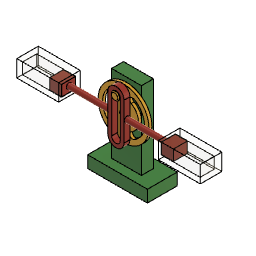
scotch yoke mechanism (piston) (Autodesk Fusion 360 design; units mm, degrees)
Autodesk Fusion 360 part; units mm, degrees
sketch "base" plane through (0, 0, 0) normal (0, 0, 1) x (1, 0, 0)
  line L0 (0, 0) -> (100, 0)
  line L1 (100, 0) -> (100, 50)
  line L2 (100, 50) -> (0, 50)
  line L3 (0, 50) -> (0, 0)
  line L4 (50, 35) -> (75, 35)
  line L5 (75, 35) -> (75, 15)
  line L6 (75, 15) -> (50, 15)
  line L7 (50, 15) -> (50, 35)
  line L8 (50, 35) -> (25, 35)
  line L9 (25, 35) -> (25, 15)
  line L10 (25, 15) -> (50, 15)
  dimension "d1" = 100
  dimension "d2" = 50
  constraint horizontal L0
  constraint vertical L1
  constraint horizontal L2
  constraint vertical L3
  constraint coincident L0.start L3.end
  constraint horizontal L4
  constraint vertical L5
  constraint horizontal L6
  constraint vertical L7
  constraint symmetric L4.start L7 L8.start
  constraint symmetric L4.end L7 L8.end
  constraint symmetric L5.end L7 L9.end
  constraint symmetric L6.end L7 L10.end
  measures "d1" distance of L0.start L0.end
  measures "d2" distance of L0.start L2.end
  measures "d85" distance of L0.start
extrude "Extrude1" add sketch "base" along normal blind 20 makes body 1
extrude "Extrude2" add sketch "base" along normal blind 150 separate body contours L4 L5 L6 L7 | L7 L8 L9 L10 makes body 2
sketch "stand" plane through (0, 15, 0) normal (0, -1, 0) x (1, 0, 0)
  line L0 (25, 0) -> (75, 0)
  line L1 (75, 0) -> (75, 150)
  line L2 (75, 150) -> (25, 150)
  line L3 (25, 150) -> (25, 0)
  circle A0 centre (50, 100) radius 5
  dimension "d7" = 10
  measures "d7" diameter of A0
extrude "Extrude3" add sketch "stand" along normal blind 7 contours A0 bodies 2
sketch "crank" plane through (0, 15, 0) normal (0, -1, 0) x (1, 0, 0)
  circle A0 centre (50, 100) radius 5
  line L0 (25, 0) -> (75, 0)
  line L1 (75, 0) -> (75, 150)
  line L2 (75, 150) -> (25, 150)
  line L3 (25, 150) -> (25, 0)
  circle A1 centre (50, 100) radius 42.5
  dimension "d10" = 85
  constraint concentric A0 A1
  measures "d10" diameter of A1
extrude "Extrude4" add sketch "crank" along normal blind 5 separate body contours L3 A1 | L1 L3 A1 | L1 A1 makes body 3
move_face "OffsetFaces1" offset -0.4 1 faces at (54.9752, 12.6667, 100.4978) on bodies 2
sketch "slots" plane through (0, 10, 0) normal (0, -1, 0) x (1, 0, 0)
  circle A0 centre (50, 100) radius 5
  circle A1 centre (50, 100) radius 42.5
  arc A2 (37.3529, 120.5882) -> (37.3529, 79.4118) centre (48.3333, 100) ccw
  arc A3 (37.3529, 120.5882) -> (32.6471, 129.4118) centre (35, 125) ccw
  arc A4 (32.6471, 129.4118) -> (32.6471, 70.5882) centre (48.3333, 100) ccw
  arc A5 (32.6471, 70.5882) -> (37.3529, 79.4118) centre (35, 75) ccw
  arc A6 (35, 125) -> (35, 75) centre (48.3333, 100) ccw construction
  line L0 (50, 142.5) -> (50, 57.5)
  arc A7 (62.6471, 79.4118) -> (62.6471, 120.5882) centre (51.6667, 100) ccw
  arc A8 (67.3529, 70.5882) -> (67.3529, 129.4118) centre (51.6667, 100) ccw
  arc A9 (67.3529, 129.4118) -> (62.6471, 120.5882) centre (65, 125) ccw
  arc A10 (62.6471, 79.4118) -> (67.3529, 70.5882) centre (65, 75) ccw
  arc A11 (65, 75) -> (65, 125) centre (51.6667, 100) ccw construction
  constraint tangent A2 A3
  constraint tangent A3 A4
  constraint tangent A4 A5
  constraint tangent A2 A5
  constraint coincident A1 L0.start
  constraint coincident A1 L0.end
  constraint vertical L0
  constraint symmetric A2.end L0 A7.start
  constraint symmetric A2.start L0 A7.end
  constraint symmetric A3.end L0 A8.end
  constraint symmetric A4.end L0 A8.start
  constraint symmetric A2 L0 A7
  constraint symmetric A3 L0 A9
  constraint symmetric A4 L0 A8
  constraint symmetric A5 L0 A10
  constraint symmetric A6 L0 A11
extrude "Extrude5" cut sketch "slots" against normal blind 5 contours A2 A3 A4 A5 | A7 A8 A9 A10 bodies 3
sketch "pin" plane through (0, 10, 0) normal (0, -1, 0) x (1, 0, 0)
  arc A0 (32.6471, 129.4118) -> (32.6471, 70.5882) centre (48.3333, 100) ccw
  arc A1 (37.3529, 120.5882) -> (32.6471, 129.4118) centre (35, 125) ccw
  arc A2 (37.3529, 120.5882) -> (37.3529, 79.4118) centre (48.3333, 100) ccw
  arc A3 (32.6471, 70.5882) -> (37.3529, 79.4118) centre (35, 75) ccw
  arc A4 (67.3529, 70.5882) -> (67.3529, 129.4118) centre (51.6667, 100) ccw
  arc A5 (62.6471, 79.4118) -> (67.3529, 70.5882) centre (65, 75) ccw
  arc A6 (62.6471, 79.4118) -> (62.6471, 120.5882) centre (51.6667, 100) ccw
  arc A7 (67.3529, 129.4118) -> (62.6471, 120.5882) centre (65, 125) ccw
  circle A8 centre (50, 100) radius 5
  circle A9 centre (50, 100) radius 42.5
  circle A10 centre (50, 132.0072) radius 6.7715
extrude "Extrude6" add sketch "pin" along normal blind 15 contours A10 bodies 3
fillet "Fillet1" radius 1.5 1 edges at (43.6867, -5, 129.5585) on bodies 3
sketch "big slot" plane through (0, 10, 0) normal (0, -1, 0) x (1, 0, 0)
  circle A0 centre (50, 132.0072) radius 6.7715
  arc A1 (32.6471, 129.4118) -> (32.6471, 70.5882) centre (48.3333, 100) ccw
  arc A2 (37.3529, 120.5882) -> (32.6471, 129.4118) centre (35, 125) ccw
  arc A3 (37.3529, 120.5882) -> (37.3529, 79.4118) centre (48.3333, 100) ccw
  arc A4 (32.6471, 70.5882) -> (37.3529, 79.4118) centre (35, 75) ccw
  arc A5 (67.3529, 70.5882) -> (67.3529, 129.4118) centre (51.6667, 100) ccw
  arc A6 (62.6471, 79.4118) -> (67.3529, 70.5882) centre (65, 75) ccw
  arc A7 (62.6471, 79.4118) -> (62.6471, 120.5882) centre (51.6667, 100) ccw
  arc A8 (67.3529, 129.4118) -> (62.6471, 120.5882) centre (65, 125) ccw
  circle A9 centre (50, 100) radius 5
  circle A10 centre (50, 100) radius 42.5
  line L0 (36.5, 132.0072) -> (36.5, 70)
  arc A11 (36.5, 70) -> (63.5, 70) centre (50, 70) ccw
  line L1 (63.5, 70) -> (63.5, 132.0072)
  arc A12 (63.5, 132.0072) -> (36.5, 132.0072) centre (50, 132.0072) ccw
  line L2 (50, 132.0072) -> (50, 70) construction
  line L3 (42.85, 132.0072) -> (42.85, 70)
  arc A13 (42.85, 70) -> (57.15, 70) centre (50, 70) ccw
  line L4 (57.15, 70) -> (57.15, 132.0072)
  arc A14 (57.15, 132.0072) -> (42.85, 132.0072) centre (50, 132.0072) ccw
  line L5 (50, 132.0072) -> (50, 70) construction
  dimension "d19" = 27
  dimension "d20" = 14.3
  constraint tangent L0 A11
  constraint tangent A11 L1
  constraint parallel L0 L1
  constraint tangent L1 A12
  constraint tangent L0 A12
  constraint vertical L2
  constraint coincident A0.centre A12.centre
  constraint tangent L3 A13
  constraint tangent A13 L4
  constraint parallel L3 L4
  constraint tangent L4 A14
  constraint tangent L3 A14
  constraint coincident A11.centre L2.end
  constraint parallel L2 L5
  measures "d19" diameter of A11
  measures "d20" diameter of A13
extrude "Extrude7" add sketch "big slot" along normal blind 10 separate body contours A2 A3 A4 A6 A7 A8 A10 L0 A11 L1 A12 | A2 A3 L0 | A3 A4 L0 | A10 A12 | A10 A11 | A7 A8 L1 | A6 A7 L1 makes body 4
move_body "Move1" bodies 4 to x (1, 0, 0) y (0, 1, 0) z (0, 0, 1) at (0, -1, 0)
sketch "arm r" plane through (63.5, 0, 0) normal (1, 0, 0) x (0, 1, 0)
  line L0 (9, 70) -> (9, 132.0072)
  line L1 (9, 132.0072) -> (-1, 132.0072)
  line L2 (-1, 132.0072) -> (-1, 70)
  line L3 (-1, 70) -> (9, 70)
  line L4 (4, 132.0072) -> (4, 102.0072)
  circle A0 centre (4, 102.0072) radius 4.5
  dimension "d23" = 30
  dimension "d24" = 9
  constraint midpoint L1 L4.start
  constraint perpendicular L3 L4
  constraint coincident L4.end A0.centre
  measures "d23" distance of L4.start L4.end
  measures "d24" diameter of A0
sketch "arm l" plane through (36.5, 0, 0) normal (-1, 0, 0) x (0, -1, 0)
  line L0 (-9, 132.0072) -> (-9, 70)
  line L1 (-9, 70) -> (1, 70)
  line L2 (1, 70) -> (1, 132.0072)
  line L3 (1, 132.0072) -> (-9, 132.0072)
  line L4 (-4, 132.0072) -> (-4, 102.0072)
  circle A0 centre (-4, 102.0072) radius 4.5
  dimension "d27" = 30
  dimension "d28" = 9
  constraint midpoint L3 L4.start
  constraint perpendicular L3 L4
  constraint coincident L4.end A0.centre
  measures "d27" distance of L4.start L4.end
  measures "d28" diameter of A0
extrude "Extrude9" add sketch "arm l" along normal blind 70 contours A0 bodies 4
extrude "Extrude10" add sketch "arm r" along normal blind 70 contours A0 bodies 4
move_body "Move2" bodies 4 to x (1, 0, 0) y (0, 1, 0) z (0, 0, 1) at (0, -1.7, 0)
sketch "slider stand" plane through (0, 0, 150) normal (0, 0, 1) x (-1, 0, 0)
  line L0 (-75, -35) -> (-25, -35)
  line L1 (-25, -35) -> (-25, -15)
  line L2 (-25, -15) -> (-75, -15)
  line L3 (-75, -15) -> (-75, -35)
  line L4 (-50, -35) -> (-77.5, -35)
  line L5 (-77.5, -35) -> (-77.5, -15)
  line L6 (-77.5, -15) -> (-50, -15)
  line L7 (-50, -15) -> (-50, -35)
  line L8 (-50, -35) -> (-22.5, -35)
  line L9 (-22.5, -15) -> (-50, -15)
  line L10 (-22.5, -35) -> (-22.5, -15)
  dimension "d33" = 27.5
  dimension "d34" = 20
  constraint horizontal L4
  constraint vertical L5
  constraint horizontal L6
  constraint vertical L7
  constraint midpoint L0 L4.start
  constraint symmetric L4.start L7 L8.start
  constraint symmetric L4.end L7 L8.end
  constraint symmetric L5.end L7 L9.start
  constraint symmetric L6.end L7 L9.end
  measures "d33" distance of L4.start L4.end
  measures "d34" distance of L4.start L6.end
sketch "slider extrusion" plane through (0, 27.5, 0) normal (0, -1, 0) x (1, 0, 0)
  line L0 (22.5, 150) -> (77.5, 150)
  line L1 (77.5, 150) -> (77.5, 175)
  line L2 (77.5, 175) -> (22.5, 175)
  line L3 (22.5, 175) -> (22.5, 150)
  line L4 (22.5, 175) -> (77.5, 175)
  line L5 (77.5, 175) -> (77.5, 170)
  line L6 (77.5, 170) -> (22.5, 170)
  line L7 (22.5, 170) -> (22.5, 175)
  line L8 (22.5, 162.5) -> (77.5, 162.5)
  line L9 (22.5, 150) -> (77.5, 150)
  line L10 (77.5, 155) -> (22.5, 155)
  line L11 (22.5, 155) -> (22.5, 150)
  line L12 (77.5, 150) -> (77.5, 155)
  dimension "d39" = 5
  constraint horizontal L4
  constraint vertical L5
  constraint horizontal L6
  constraint vertical L7
  constraint coincident L1 L5.end
  constraint coincident L2.end L3.start
  constraint midpoint L3 L8.start
  constraint midpoint L1 L8.end
  constraint symmetric L2.end L8 L0.start
  constraint symmetric L1.end L8 L0.end
  constraint symmetric L5.end L8 L10.start
  constraint symmetric L6.end L8 L10.end
  measures "d39" distance of L2.end L6.end
sketch "slider support up" plane through (0, 0, 170) normal (0, 0, -1) x (1, 0, 0)
  line L0 (77.5, -27.5) -> (77.5, -15)
  line L1 (77.5, -15) -> (22.5, -15)
  line L2 (22.5, -15) -> (22.5, -27.5)
  line L3 (22.5, -15) -> (77.5, -15)
  line L4 (77.5, -15) -> (77.5, -18)
  line L5 (77.5, -18) -> (22.5, -18)
  line L6 (22.5, -18) -> (22.5, -15)
  line L7 (22.5, -27.5) -> (77.5, -27.5)
  dimension "d42" = 3
  constraint horizontal L3
  constraint vertical L4
  constraint horizontal L5
  constraint vertical L6
  constraint coincident L1.end L2.start
  measures "d42" distance of L1.end L5.end
sketch "slider support down" plane through (0, 0, 155) normal (0, 0, 1) x (-1, 0, 0)
  line L0 (-22.5, -27.5) -> (-22.5, -15)
  line L1 (-22.5, -15) -> (-77.5, -15)
  line L2 (-77.5, -15) -> (-77.5, -27.5)
  line L3 (-22.5, -15) -> (-77.5, -15)
  line L4 (-77.5, -15) -> (-77.5, -18)
  line L5 (-77.5, -18) -> (-22.5, -18)
  line L6 (-22.5, -18) -> (-22.5, -15)
  line L7 (-77.5, -27.5) -> (-22.5, -27.5)
  dimension "d43" = 3
  constraint horizontal L3
  constraint vertical L4
  constraint horizontal L5
  constraint vertical L6
  constraint coincident L0.end L1.start
  measures "d43" distance of L0.end L5.end
sketch "slider" plane through (77.5, 0, 0) normal (1, 0, 0) x (0, 1, 0)
  line L0 (18, 155) -> (18, 159)
  line L1 (18, 159) -> (15, 159)
  line L2 (15, 159) -> (15, 155)
  line L3 (18, 170) -> (27.5, 170)
  line L4 (27.5, 170) -> (27.5, 155)
  line L5 (27.5, 155) -> (18, 155)
  line L6 (18, 155) -> (18, 170)
  line L7 (15, 155) -> (18, 155)
  constraint horizontal L3
  constraint vertical L4
  constraint horizontal L5
  constraint vertical L6
sketch "slider arms down" plane through (0, 0, 155) normal (0, 0, -1) x (1, 0, 0)
  line L0 (-40.5, -27.5) -> (-33.5, -27.5)
  line L1 (-33.5, -18) -> (-40.5, -18)
  line L2 (-40.5, -18) -> (-40.5, -27.5)
  line L3 (-40.5, -18) -> (-33.5, -18)
  line L4 (-33.5, -18) -> (-33.5, -27.5)
  line L5 (-33.5, -27.5) -> (-40.5, -27.5)
  line L6 (-40.5, -27.5) -> (-40.5, -18)
  line L7 (-33.5, -18) -> (-40.5, -18)
  line L8 (-40.5, -18) -> (-40.5, -27.5)
  line L9 (-40.5, -27.5) -> (-33.5, -27.5)
  line L10 (-33.5, -27.5) -> (-33.5, -18)
  line L11 (-33.5, -27.5) -> (-33.5, -18)
  dimension "d56" = 7
  dimension "d57" = 7
  constraint horizontal L3
  constraint vertical L4
  constraint horizontal L5
  constraint vertical L6
  constraint coincident L1.end L2.start
  constraint horizontal L7
  constraint vertical L8
  constraint horizontal L9
  constraint vertical L10
  constraint coincident L1.start L3.end
  measures "d56" distance of L1.end L1.start
  measures "d57" distance of L1.start L1.end
sketch "slider arms front" plane through (0, 18, 0) normal (0, -1, 0) x (1, 0, 0)
  line L0 (-40.5, 155) -> (-40.5, 97.55)
  line L1 (-40.5, 97.55) -> (-33.5, 97.55)
  line L2 (-40.5, 97.55) -> (-33.5, 97.55)
  line L3 (-33.5, 97.55) -> (-33.5, 106.55)
  line L4 (-33.5, 106.55) -> (-40.5, 106.55)
  line L5 (-40.5, 106.55) -> (-40.5, 97.55)
  line L6 (140.5, 97.55) -> (133.5, 97.55)
  line L7 (133.5, 97.55) -> (133.5, 106.55)
  line L8 (133.5, 106.55) -> (140.5, 106.55)
  line L9 (140.5, 106.55) -> (140.5, 97.55)
  line L10 (-33.5, 97.55) -> (-33.5, 155)
  line L11 (-33.5, 155) -> (-40.5, 155)
  dimension "d60" = 9
  dimension "d61" = 9
  constraint horizontal L2
  constraint vertical L3
  constraint horizontal L4
  constraint vertical L5
  constraint coincident L0.end L1.start
  constraint horizontal L6
  constraint vertical L7
  constraint horizontal L8
  constraint vertical L9
  measures "d60" distance of L0.end L4.end
  measures "d61" distance of L6.start L8.end
copy_body "Body->Comp1" bodies 1 removing the originals makes body 5 in component "base"
copy_body "Body->Comp2" bodies 2 removing the originals makes body 6 in component "stand"
copy_body "Body->Comp3" bodies 3 removing the originals makes body 7 in component "crank"
copy_body "Body->Comp4" bodies 4 removing the originals makes body 8 in component "slot with arms"
sketch "Sketch18" plane through (133.5, 0, 0) normal (1, 0, 0) x (0, 1, 0)
  circle A0 centre (2.3, 102.0072) radius 4.5
  line L0 (-10, 110) -> (13, 110)
  line L1 (13, 110) -> (13, 92)
  line L2 (13, 92) -> (-10, 92)
  line L3 (-10, 92) -> (-10, 110)
  constraint horizontal L0
  constraint vertical L1
  constraint horizontal L2
  constraint vertical L3
sketch "Sketch19" plane through (-33.5, 0, 0) normal (-1, 0, 0) x (0, -1, 0)
  circle A0 centre (-2.3, 102.0072) radius 4.5
  line L0 (10, 110) -> (-13, 110)
  line L1 (-13, 110) -> (-13, 92)
  line L2 (-13, 92) -> (10, 92)
  line L3 (10, 92) -> (10, 110)
  dimension "d74" = 23
  dimension "d75" = 18
  constraint horizontal L0
  constraint vertical L1
  constraint horizontal L2
  constraint vertical L3
  measures "d74" distance of L0.start L0.end
  measures "d75" distance of L0.start L2.end
extrude "Extrude1'" add sketch "Sketch18" along normal blind 20 contours A0 | L0 L1 L2 L3 bodies 8 in component "slot with arms"
extrude "Extrude2'" add sketch "Sketch19" along normal blind 20 contours A0 | L0 L1 L2 L3 bodies 8 in component "slot with arms"
sketch "Sketch20" plane through (-33.5, 0, 0) normal (-1, 0, 0) x (0, -1, 0)
  circle A0 centre (-2.3, 102.0072) radius 4.5
  line L0 (10, 110) -> (-13, 110)
  line L1 (-13, 110) -> (-13, 92)
  line L2 (-13, 92) -> (10, 92)
  line L3 (10, 92) -> (10, 110)
  line L4 (15, 115) -> (-21, 115)
  line L5 (-21, 115) -> (-21, 87)
  line L6 (-21, 87) -> (15, 87)
  line L7 (15, 87) -> (15, 115)
  dimension "d80" = 23
  dimension "d81" = 18
  dimension "d82" = 36
  dimension "d83" = 28
  constraint horizontal L0
  constraint vertical L1
  constraint horizontal L2
  constraint vertical L3
  constraint horizontal L4
  constraint vertical L5
  constraint horizontal L6
  constraint vertical L7
  measures "d80" distance of L0.start L0.end
  measures "d81" distance of L0.start L2.end
  measures "d82" distance of L4.start L4.end
  measures "d83" distance of L4.start L6.end
sketch "Sketch21" plane through (133.5, 0, 0) normal (1, 0, 0) x (0, 1, 0)
  circle A0 centre (2.3, 102.0072) radius 4.5
  line L0 (-10, 110) -> (13, 110)
  line L1 (13, 110) -> (13, 92)
  line L2 (13, 92) -> (-10, 92)
  line L3 (-10, 92) -> (-10, 110)
  line L4 (-15, 115) -> (21, 115)
  line L5 (21, 115) -> (21, 87)
  line L6 (21, 87) -> (-15, 87)
  line L7 (-15, 87) -> (-15, 115)
  dimension "d84" = 23
  dimension "d85" = 18
  dimension "d86" = 36
  dimension "d87" = 28
  constraint horizontal L0
  constraint vertical L1
  constraint horizontal L2
  constraint vertical L3
  constraint horizontal L4
  constraint vertical L5
  constraint horizontal L6
  constraint vertical L7
  measures "d84" distance of L0.start L0.end
  measures "d85" distance of L0.start L2.end
  measures "d86" distance of L4.start L4.end
  measures "d87" distance of L4.start L6.end
extrude "Extrude22" add sketch "Sketch21" along normal blind 70 separate body contours L4 L5 L6 L7 makes body 9
extrude "Extrude23" add sketch "Sketch20" along normal blind 70 separate body contours L4 L5 L6 L7 makes body 10
extrude "Extrude24" add sketch "Sketch19" along normal blind 70 contours A0 | L0 L1 L2 L3 bodies 10
extrude "Extrude25" cut sketch "Sketch19" along normal blind 65 contours A0 | L0 L1 L2 L3 bodies 10
extrude "Extrude26" add sketch "Sketch18" along normal blind 70 contours A0 | L0 L1 L2 L3 bodies 9
extrude "Extrude27" cut sketch "Sketch18" along normal blind 65 contours A0 | L0 L1 L2 L3 bodies 9
move_face "OffsetFaces2" offset -0.3 4 faces at (-55.1667, 13, 104) (-55.1667, -2.3333, 110) (-55.1667, 5.3333, 92) (-55.1667, -10, 98) on bodies 10
move_face "OffsetFaces3" offset -0.3 4 faces at (155.1667, 13, 104) (155.1667, 5.3333, 92) (155.1667, -10, 98) (155.1667, -2.3333, 110) on bodies 9
copy_body "Body->Comp7" bodies 9 removing the originals makes body 11 in component "piston right"
copy_body "Body->Comp8" bodies 10 removing the originals makes body 12 in component "piston left"
component "base" placed x (1, 0, 0) y (0, 1, 0) z (0, 0, 1) at (0, 0, 0)
component "stand" placed x (1, 0, 0) y (0, 1, 0) z (0, 0, 1) at (0, 0, 0)
component "crank" placed x (1, 0, 0) y (0, 1, 0) z (0, 0, 1) at (0, 0, 0)
component "slot with arms" placed x (1, 0, 0) y (0, 1, 0) z (0, 0, 1) at (0, 0, 0)
component "piston right" placed x (1, 0, 0) y (0, 1, 0) z (0, 0, 1) at (0, 0, 0)
component "piston left" placed x (1, 0, 0) y (0, 1, 0) z (0, 0, 1) at (0, 0, 0)
named bodies: "base", "stand", "crank", "slot with arms"
